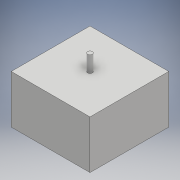
# Autodesk Inventor part: moteur
Saved by Autodesk Inventor 2017 (Build 210142000, 142)
## iProperties
Created: 2017-11-16
Part Number: moteur
Material: Generic
Document SubType Name: Modeling
Designer: Biscuit
Density: 1 g/cm^3
Appearance: Default
Author: Biscuit
Autodesk Inventor part; units mm, degrees
ref_plane "YZ Plane" through (0, 0, 0) normal (1, 0, 0) x (0, 1, 0)
ref_plane "XZ Plane" through (0, 0, 0) normal (0, 1, 0) x (-1, 0, 0)
ref_plane "XY Plane" through (0, 0, 0) normal (0, 0, 1) x (1, 0, 0)
sketch "Sketch1" plane through (0, 0, 0) normal (0, 0, 1) x (1, 0, 0)
  line L0 (0, 0) -> (49, 0)
  line L1 (49, 0) -> (49, 49)
  line L2 (49, 49) -> (0, 49)
  line L3 (0, 49) -> (0, 0)
  dimension "d0" = 49
  dimension "d1" = 49
  constraints: 8 end point, 2 parallel, 1 horizontal, 1 perpendicular
  measures "d0" distance of L1.end L2.end
  measures "d1" distance of L2.end L0.start
extrude "Extrusion1" add sketch "Sketch1" along normal blind 30
sketch "Sketch2" plane through (0, 0, 30) normal (0, 0, 1) x (1, 0, 0)
  circle A0 centre (24.5, 24.5) radius 1.5
  line L0 (49, 49) -> (0, 49) projected
  line L1 (0, 0) -> (49, 0) projected
  line L2 (49, 0) -> (49, 49) projected
  line L3 (0, 49) -> (0, 0) projected
  dimension "d4" = 3
  dimension "d5" = 49
  dimension "d6" = 49
  dimension "d7" = 24.5
  dimension "d8" = 24.5
  constraints: 1 centre point
  measures "d4" diameter of A0
  measures "d5" distance between parallel lines of L0 L1
  measures "d6" distance between parallel lines of L2 L3
  measures "d7" distance from line of L2 A0.centre
  measures "d8" distance from line of L0 A0.centre
extrude "Extrusion2" add sketch "Sketch2" along normal blind 10 contours A0
equation "\"d7\" = 0.5 * d6"
equation "\"d8\" = 0.5 * d5"
body "Solid1"
